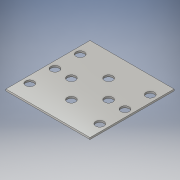
# Autodesk Inventor part: goniometer_stage_shim_v1
Saved by Autodesk Inventor 2016 (Build 200138000, 138)
## iProperties
Created: 2017-01-09
Part Number: goniometer_stage_shim_v1
Material: Stainless Steel AISI 304
Document SubType Name: Modeling
Designer: stephenholtz
Density: 8 g/cm^3
Appearance: Chrome - Satin
Author: stephenholtz
Autodesk Inventor part; units mm, degrees
ref_plane "YZ Plane" through (0, 0, 0) normal (1, 0, 0) x (0, 1, 0)
ref_plane "XZ Plane" through (0, 0, 0) normal (0, 1, 0) x (-1, 0, 0)
ref_plane "XY Plane" through (0, 0, 0) normal (0, 0, 1) x (1, 0, 0)
sketch "adapter-hole-geometry" plane through (0, 0, 0) normal (0, 0, 1) x (1, 0, 0)
  line L0 (15.875, -11.43) -> (-15.875, -11.43) construction
  line L1 (-15.875, -11.43) -> (-15.875, 11.43) construction
  line L2 (-15.875, 11.43) -> (15.875, 11.43) construction
  line L3 (15.875, 11.43) -> (15.875, -11.43) construction
  line L4 (15.875, -11.43) -> (-15.875, 11.43) construction
  line L5 (-15.875, -11.43) -> (15.875, 11.43) construction
  line L6 (11.43, -15.875) -> (-11.43, -15.875) construction
  line L7 (-11.43, -15.875) -> (-11.43, 15.875) construction
  line L8 (-11.43, 15.875) -> (11.43, 15.875) construction
  line L9 (11.43, 15.875) -> (11.43, -15.875) construction
  line L10 (11.43, -15.875) -> (-11.43, 15.875) construction
  line L11 (-11.43, -15.875) -> (11.43, 15.875) construction
  line L12 (0, -8.4414) -> (8.4414, 0) construction
  line L13 (8.4414, 0) -> (0, 8.4414) construction
  line L14 (0, 8.4414) -> (-8.4414, 0) construction
  line L15 (-8.4414, 0) -> (0, -8.4414) construction
  line L16 (-5.969, -5.969) -> (5.969, 5.969) construction
  line L17 (5.969, -5.969) -> (-5.969, 5.969) construction
  line L18 (-8.4414, -8.4414) -> (8.4414, -8.4414) construction
  line L19 (8.4414, -8.4414) -> (8.4414, 8.4414) construction
  line L20 (8.4414, 8.4414) -> (-8.4414, 8.4414) construction
  line L21 (-8.4414, 8.4414) -> (-8.4414, -8.4414) construction
  line L22 (-8.4414, -8.4414) -> (8.4414, 8.4414) construction
  line L23 (8.4414, -8.4414) -> (-8.4414, 8.4414) construction
  point P0 (0, 0)
  point P1 (0, 8.4414)
  point P2 (8.4414, 0)
  dimension "d29" = 31.75
  dimension "d30" = 22.86
  dimension "d31" = 22.86
  dimension "d32" = 31.75
  dimension "d33" = 11.938
  dimension "d34" = 11.938
  dimension "d42" = 16.8829
  dimension "d43" = 16.8829
  dimension "d58" = 4.445
  dimension "d59" = 7.4336
  dimension "d60" = 5.969
  dimension "d61" = 5.969
  dimension "d62" = 4.445
  dimension "d63" = 7.4336
  dimension "d64" = 9.906
  dimension "d65" = 9.906
  dimension "d66" = 15.875
  dimension "d67" = 5.969
  dimension "d68" = 21.844
  dimension "d69" = 21.844
  measures "d29" distance of L1.end L2.end
  measures "d30" distance of L0.end L1.end
  measures "d31" distance of L7.end L8.end
  measures "d32" distance of L6.end L7.end
  measures "d33" distance of L14.end L13.end
  measures "d34" distance of L13.end L12.end
  measures "d42" distance between parallel lines of L18 L20
  measures "d43" distance between parallel lines of L21 L19
  measures "d58" distance between parallel lines of L3 L9
  measures "d59" distance between parallel lines of L3 L19
  measures "d60" distance between parallel lines of L17 L13
  measures "d61" distance between parallel lines of L16 L12
  measures "d62" distance between parallel lines of L2 L8
  measures "d63" distance between parallel lines of L8 L20
  measures "d64" distance from line of L16.end L3
  measures "d65" distance from line of L17.start L3
  measures "d66" distance from line of point (0, 0) L3
  measures "d67" distance from line of point (0, 0) L13
  measures "d68" distance from line of L17.end L3
  measures "d69" distance from line of L16.start L3
sketch "Sketch1" plane through (0, 0, 0) normal (0, 0, 1) x (1, 0, 0)
  line L0 (19.05, -19.05) -> (-19.05, -19.05)
  line L1 (-19.05, -19.05) -> (-19.05, 19.05)
  line L2 (-19.05, 19.05) -> (19.05, 19.05)
  line L3 (19.05, 19.05) -> (19.05, -19.05)
  line L4 (19.05, -19.05) -> (-19.05, 19.05) construction
  line L5 (-19.05, -19.05) -> (19.05, 19.05) construction
  point P0 (0, 0)
  dimension "d0" = 38.1
  dimension "d1" = 38.1
  constraints: 12 end point, 2 midpoint, 2 parallel, 1 horizontal, 1 perpendicular
  measures "d0" distance of L1.end L2.end
  measures "d1" distance of L0.end L1.end
extrude "Extrusion1" add sketch "Sketch1" along normal blind 0.7937
sketch "Sketch4" plane through (0, 0, 0.7937) normal (0, 0, 1) x (1, 0, 0)
  line L0 (-19.05, -19.05) -> (19.05, -19.05) construction
  line L1 (19.05, -19.05) -> (19.05, 19.05) construction
  line L2 (19.05, 19.05) -> (-19.05, 19.05) construction
  line L3 (-19.05, 19.05) -> (-19.05, -19.05) construction
  point P0 (0, 0)
  point P1 (-15.875, 11.43)
  point P2 (-15.875, 0)
  point P3 (-15.875, -11.43)
  point P4 (15.875, -11.43)
  point P5 (15.875, 0)
  point P6 (15.875, 11.43)
  point P7 (0, 8.4414)
  point P8 (-8.4414, 0)
  point P9 (0, -8.4414)
  point P10 (8.4414, 0)
  dimension "d44" = 3.175
  dimension "d45" = 3.175
  dimension "d46" = 7.62
  dimension "d47" = 3.175
  dimension "d48" = 7.62
  dimension "d49" = 3.175
  dimension "d50" = 7.62
  constraints: 18 other
hole "Hole3" at (-15.875, 11.43, 0.7937) at (-15.875, 0, 0.7937) at (-15.875, -11.43, 0.7937) at (15.875, -11.43, 0.7937) at (15.875, 0, 0.7937) at (15.875, 11.43, 0.7937) at (0, 8.4414, 0.7937) at (-8.4414, 0, 0.7937) at (0, -8.4414, 0.7937) at (8.4414, 0, 0.7937) direction (0, 0, -1) diameter 3.7973 end through all
body "Solid1"
